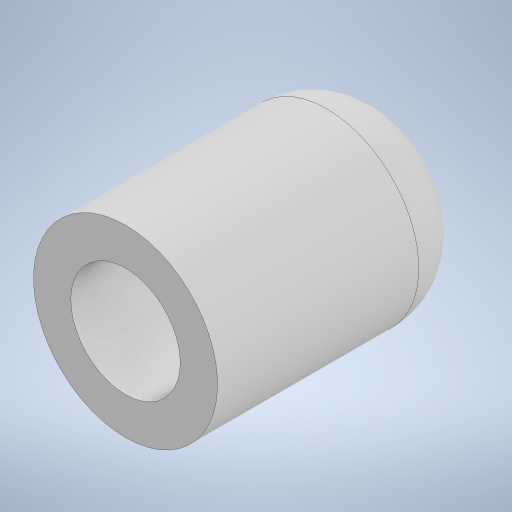
# Autodesk Inventor part: Задание номер 12
Saved by Autodesk Inventor 2023.2 (Build 272271030, 271C)
## iProperties
Created: 2023-09-07
Part Number: Задание номер 12
Material: Типовые
Document SubType Name: Modeling
Designer: User
Density: 1 g/cm^3
Appearance: По умолчанию
Author: User
Autodesk Inventor part; units mm, degrees
ref_plane "YZ Plane" through (0, 0, 0) normal (1, 0, 0) x (0, 1, 0)
ref_plane "XZ Plane" through (0, 0, 0) normal (0, 1, 0) x (-1, 0, 0)
ref_plane "XY Plane" through (0, 0, 0) normal (0, 0, 1) x (1, 0, 0)
sketch "Эскиз1" plane through (0, 0, 0) normal (1, 0, 0) x (0, 1, 0)
  line L0 (-2.2145, -6.8214) -> (-2.2145, 3.9786)
  arc A0 (-2.2145, -6.8214) -> (0.9855, -10.0214) centre (0.9855, -6.8214) ccw
  line L1 (2.7225, -8.0214) -> (2.7225, 3.9786)
  line L2 (-0.2145, 3.9786) -> (-0.2145, -3.8549)
  line L3 (-0.2145, -3.8549) -> (-0.2145, -6.2214)
  line L4 (-0.2145, -6.2214) -> (-0.2145, -6.5844)
  line L5 (1.5855, -8.0214) -> (1.2225, -8.0214)
  arc A1 (-0.2145, -6.5844) -> (1.2225, -8.0214) centre (1.2225, -6.5844) ccw
  line L6 (2.7225, -8.0214) -> (2.7225, 3.9786)
  line L7 (1.2225, -8.0214) -> (1.2225, -10.0214)
  line L8 (1.2225, -10.0214) -> (0.9855, -10.0214)
  line L9 (-0.2145, 3.9786) -> (-2.2145, 3.9786)
  point P0 (1.2855, -8.0214)
  dimension "d1" = 3.2
  dimension "d3" = 14
  dimension "d9" = 2
  dimension "d14" = 1.437
  dimension "d16" = 1.5
  constraints: 20 end point, 6 vertical, 5 point on circle, 3 horizontal, 3 tangent, 2 centre point, 1 point on line
  measures "d1" radius of A0
  measures "d3" vertical distance of L0.end L8.end
  measures "d9" distance of L0.end L2.start
  measures "d14" radius of A1
  measures "d16" distance of L1.start L5.end
sketch "Эскиз2" plane through (0, 0, 0) normal (1, 0, 0) x (0, 1, 0)
  point P0 (0, 0)
sketch "Эскиз3" plane through (0, 0, 0) normal (1, 0, 0) x (0, 1, 0)
  point P0 (0, 0)
sketch "Эскиз4" plane through (0, 0, 0) normal (1, 0, 0) x (0, 1, 0)
  point P0 (0, 0)
revolve "Вращение1" add sketch "Эскиз1" angle 360 about axis through (0, 2.7225, -8.0214) along (0, 0, 1)
